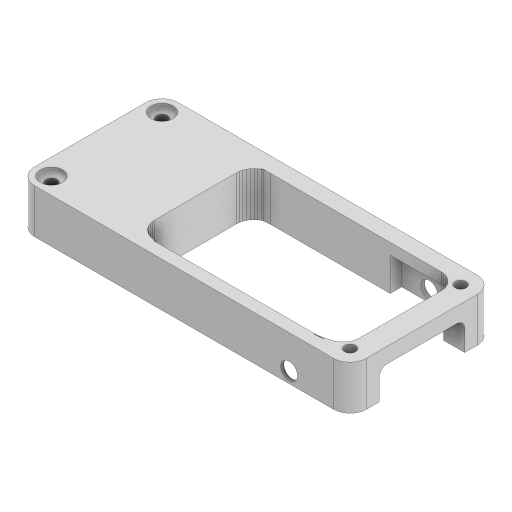
# Autodesk Inventor part: atas
Saved by Autodesk Inventor 2023 (Build 270158000, 158)
## iProperties
Created: 2025-11-27
Part Number: atas
Material: Generic
Document SubType Name: Modeling
Designer: dinoo
Density: 1 g/cm^3
Appearance: Default
Author: dinoo
Autodesk Inventor part; units mm, degrees
ref_plane "YZ Plane" through (0, 0, 0) normal (1, 0, 0) x (0, 1, 0)
ref_plane "XZ Plane" through (0, 0, 0) normal (0, 1, 0) x (-1, 0, 0)
ref_plane "XY Plane" through (0, 0, 0) normal (0, 0, 1) x (1, 0, 0)
sketch "Sketch1" plane through (0, 0, 0) normal (0, 1, 0) x (-1, 0, 0)
  circle A0 centre (50.1877, 0.0488) radius 1
  circle A1 centre (-3.8123, 20.0488) radius 1
  circle A2 centre (50.1877, 20.0488) radius 1
  circle A3 centre (-3.8123, 0.0488) radius 1
  arc A4 (53.1877, 20.0488) -> (50.1877, 23.0488) centre (50.1877, 20.0488) ccw
  line L0 (50.1877, 23.0488) -> (-3.8123, 23.0488)
  arc A5 (-3.8123, 23.0488) -> (-6.8123, 20.0488) centre (-3.8123, 20.0488) ccw
  line L1 (-6.8123, 20.0488) -> (-6.8123, 0.0488)
  arc A6 (-6.8123, 0.0488) -> (-3.8123, -2.9512) centre (-3.8123, 0.0488) ccw
  line L2 (-3.8123, -2.9512) -> (50.1877, -2.9512)
  arc A7 (50.1877, -2.9512) -> (53.1877, 0.0488) centre (50.1877, 0.0488) ccw
  line L3 (53.1877, 0.0488) -> (53.1877, 20.0488)
  line L4 (-2.6184, 2.7963) -> (-2.5855, 2.3799)
  line L5 (-2.5855, 2.3799) -> (-2.4895, 1.9806)
  line L6 (-2.4895, 1.9806) -> (-2.3323, 1.6012)
  line L7 (-2.3323, 1.6012) -> (-2.1176, 1.2511)
  line L8 (-2.1176, 1.2511) -> (-1.8508, 0.9389)
  line L9 (-1.8508, 0.9389) -> (-1.5385, 0.6723)
  line L10 (-1.5385, 0.6723) -> (-1.1883, 0.4578)
  line L11 (-1.1883, 0.4578) -> (-0.8088, 0.3008)
  line L12 (-0.8088, 0.3008) -> (-0.4112, 0.2055)
  line L13 (-0.4112, 0.2055) -> (0.0053, 0.181)
  line L14 (0.0053, 0.181) -> (30.79, 0.181)
  line L15 (30.79, 0.181) -> (32.3493, 0.3042)
  line L16 (32.3493, 0.3042) -> (31.6548, 0.1372)
  line L17 (31.6548, 0.1372) -> (32.0605, 0.3054)
  line L18 (32.0605, 0.3054) -> (32.4348, 0.535)
  line L19 (32.4348, 0.535) -> (32.7687, 0.8203)
  line L20 (32.7687, 0.8203) -> (33.0538, 1.1543)
  line L21 (33.0538, 1.1543) -> (33.2832, 1.5288)
  line L22 (33.2832, 1.5288) -> (33.4511, 1.9345)
  line L23 (33.4511, 1.9345) -> (33.5535, 2.3616)
  line L24 (33.5535, 2.3616) -> (33.5792, 2.7994)
  line L25 (33.5792, 2.7994) -> (33.5837, 17.5394)
  line L26 (33.5837, 17.5394) -> (33.5491, 17.9772)
  line L27 (33.5491, 17.9772) -> (33.4465, 18.4042)
  line L28 (33.4465, 18.4042) -> (33.2783, 18.8099)
  line L29 (33.2783, 18.8099) -> (33.0488, 19.1843)
  line L30 (33.0488, 19.1843) -> (32.7635, 19.5181)
  line L31 (32.7635, 19.5181) -> (32.4294, 19.8032)
  line L32 (32.4294, 19.8032) -> (32.0549, 20.0326)
  line L33 (32.0549, 20.0326) -> (31.6492, 20.2005)
  line L34 (31.6492, 20.2005) -> (30.2225, 20.5426)
  line L35 (30.2225, 20.5426) -> (30.7843, 20.5096)
  line L36 (30.7843, 20.5096) -> (0.0014, 20.5096)
  line L37 (0.0014, 20.5096) -> (1.8279, 20.6539)
  line L38 (1.8279, 20.6539) -> (-0.8143, 20.0188)
  line L39 (-0.8143, 20.0188) -> (-1.1937, 19.8615)
  line L40 (-1.1937, 19.8615) -> (-1.5438, 19.6468)
  line L41 (-1.5438, 19.6468) -> (-1.856, 19.38)
  line L42 (-1.856, 19.38) -> (-2.1226, 19.0677)
  line L43 (-2.1226, 19.0677) -> (-2.3371, 18.7175)
  line L44 (-2.3371, 18.7175) -> (-2.4941, 18.338)
  line L45 (-2.4941, 18.338) -> (-2.5895, 17.9404)
  line L46 (-2.5895, 17.9404) -> (-2.6139, 17.5239)
  line L47 (-2.6139, 17.5239) -> (-2.6184, 2.7963)
  circle A8 centre (-0.3906, 1.9999) radius 1.125
  circle A9 centre (3.3955, 0.901) radius 0.35
  line L48 (-1.826, 5.5906) -> (-1.026, 5.5908)
  arc A10 (-1.8262, 6.0906) -> (-1.826, 5.5906) centre (-1.8261, 5.8406) ccw
  line L49 (-1.0262, 6.0908) -> (-1.8262, 6.0906)
  arc A11 (-1.026, 5.5908) -> (-1.0262, 6.0908) centre (-1.0261, 5.8408) ccw
  line L50 (2.154, 5.5917) -> (3.3539, 5.592)
  arc A12 (2.1538, 6.0917) -> (2.154, 5.5917) centre (2.1539, 5.8417) ccw
  line L51 (3.3538, 6.092) -> (2.1538, 6.0917)
  arc A13 (3.3539, 5.592) -> (3.3538, 6.092) centre (3.3539, 5.842) ccw
  circle A14 centre (5.0955, 0.9015) radius 0.35
  circle A15 centre (8.525, 1.2724) radius 0.5
  line L52 (10.5172, 4.4875) -> (10.0672, 4.4874)
  arc A16 (10.5174, 3.9375) -> (10.5172, 4.4875) centre (10.5173, 4.2125) ccw
  line L53 (10.0674, 3.9374) -> (10.5174, 3.9375)
  arc A17 (10.0672, 4.4874) -> (10.0674, 3.9374) centre (10.0673, 4.2124) ccw
  circle A18 centre (11.065, 1.2731) radius 0.5
  circle A19 centre (2.2518, 13.0567) radius 0.381
  circle A20 centre (2.2535, 7.2768) radius 0.381
  line L54 (-1.8284, 14.2406) -> (-1.0285, 14.2408)
  arc A21 (-1.8286, 14.7406) -> (-1.8284, 14.2406) centre (-1.8285, 14.4906) ccw
  line L55 (-1.0286, 14.7408) -> (-1.8286, 14.7406)
  arc A22 (-1.0285, 14.2408) -> (-1.0286, 14.7408) centre (-1.0285, 14.4908) ccw
  circle A23 centre (-0.3951, 18.3199) radius 1.125
  line L56 (2.1515, 14.2417) -> (3.3515, 14.242)
  arc A24 (2.1514, 14.7417) -> (2.1515, 14.2417) centre (2.1515, 14.4917) ccw
  line L57 (3.3514, 14.742) -> (2.1514, 14.7417)
  arc A25 (3.3515, 14.242) -> (3.3514, 14.742) centre (3.3515, 14.492) ccw
  line L58 (10.5139, 16.3375) -> (10.0639, 16.3374)
  arc A26 (10.5141, 15.7875) -> (10.5139, 16.3375) centre (10.514, 16.0625) ccw
  line L59 (10.0641, 15.7874) -> (10.5141, 15.7875)
  arc A27 (10.0639, 16.3374) -> (10.0641, 15.7874) centre (10.064, 16.0624) ccw
  circle A28 centre (3.3904, 19.4208) radius 0.35
  circle A29 centre (8.52, 19.0524) radius 0.5
  circle A30 centre (5.0904, 19.4213) radius 0.35
  circle A31 centre (18.685, 1.2752) radius 0.5
  circle A32 centre (21.225, 1.2759) radius 0.5
  circle A33 centre (13.605, 1.2738) radius 0.5
  circle A34 centre (16.145, 1.2745) radius 0.5
  circle A35 centre (23.765, 1.2767) radius 0.5
  circle A36 centre (26.305, 1.2774) radius 0.5
  circle A37 centre (28.845, 1.2781) radius 0.5
  circle A38 centre (31.609, 3.5289) radius 1.125
  circle A39 centre (16.14, 19.0545) radius 0.5
  circle A40 centre (18.68, 19.0552) radius 0.5
  circle A41 centre (11.06, 19.0531) radius 0.5
  circle A42 centre (13.6, 19.0538) radius 0.5
  circle A43 centre (28.84, 19.0581) radius 0.5
  circle A44 centre (31.6053, 16.8088) radius 1.125
  circle A45 centre (21.22, 19.0559) radius 0.5
  circle A46 centre (26.3, 19.0574) radius 0.5
  circle A47 centre (23.76, 19.0567) radius 0.5
  line L60 (33.9837, 17.5551) -> (33.9792, 2.7876)
  line L61 (33.9792, 2.7876) -> (33.9507, 2.3028)
  line L62 (33.9507, 2.3028) -> (33.8327, 1.8107)
  line L63 (33.8327, 1.8107) -> (33.6407, 1.3467)
  line L64 (33.6407, 1.3467) -> (33.3785, 0.9185)
  line L65 (33.3785, 0.9185) -> (33.0525, 0.5366)
  line L66 (33.0525, 0.5366) -> (32.6708, 0.2104)
  line L67 (32.6708, 0.2104) -> (32.2427, -0.0521)
  line L68 (32.2427, -0.0521) -> (31.7789, -0.2443)
  line L69 (31.7789, -0.2443) -> (32.4121, -0.0921)
  line L70 (32.4121, -0.0921) -> (30.8058, -0.219)
  line L71 (30.8058, -0.219) -> (-0.0064, -0.219)
  line L72 (-0.0064, -0.219) -> (-0.47, -0.1918)
  line L73 (-0.47, -0.1918) -> (-0.9327, -0.0808)
  line L74 (-0.9327, -0.0808) -> (-1.3703, 0.1003)
  line L75 (-1.3703, 0.1003) -> (-1.7742, 0.3476)
  line L76 (-1.7742, 0.3476) -> (-2.1344, 0.6551)
  line L77 (-2.1344, 0.6551) -> (-2.4421, 1.0152)
  line L78 (-2.4421, 1.0152) -> (-2.6897, 1.419)
  line L79 (-2.6897, 1.419) -> (-2.8711, 1.8565)
  line L80 (-2.8711, 1.8565) -> (-2.9818, 2.317)
  line L81 (-2.9818, 2.317) -> (-3.0184, 2.7806)
  line L82 (-3.0184, 2.7806) -> (-3.0139, 17.5357)
  line L83 (-3.0139, 17.5357) -> (-2.9867, 17.9992)
  line L84 (-2.9867, 17.9992) -> (-2.8758, 18.4619)
  line L85 (-2.8758, 18.4619) -> (-2.6946, 18.8995)
  line L86 (-2.6946, 18.8995) -> (-2.4473, 19.3034)
  line L87 (-2.4473, 19.3034) -> (-2.1398, 19.6637)
  line L88 (-2.1398, 19.6637) -> (-1.7797, 19.9714)
  line L89 (-1.7797, 19.9714) -> (-1.3759, 20.2189)
  line L90 (-1.3759, 20.2189) -> (-0.9384, 20.4003)
  line L91 (-0.9384, 20.4003) -> (1.765, 21.0502)
  line L92 (1.765, 21.0502) -> (-0.0143, 20.9096)
  line L93 (-0.0143, 20.9096) -> (30.796, 20.9096)
  line L94 (30.796, 20.9096) -> (30.2813, 20.9398)
  line L95 (30.2813, 20.9398) -> (31.773, 20.5822)
  line L96 (31.773, 20.5822) -> (32.237, 20.3901)
  line L97 (32.237, 20.3901) -> (32.6652, 20.1279)
  line L98 (32.6652, 20.1279) -> (33.0471, 19.8019)
  line L99 (33.0471, 19.8019) -> (33.3733, 19.4202)
  line L100 (33.3733, 19.4202) -> (33.6358, 18.9921)
  line L101 (33.6358, 18.9921) -> (33.8281, 18.5283)
  line L102 (33.8281, 18.5283) -> (33.9454, 18.0401)
  line L103 (33.9454, 18.0401) -> (33.9837, 17.5551)
  point P0 (0, 0)
  point P1 (-6.8123, -2.9512)
  point P2 (-2.79, -0.0008)
  point P3 (31.9888, 0.2757)
  point P4 (1.2278, 20.5096)
  point P5 (30.3601, 20.5096)
  point P6 (32.0835, -0.1181)
  point P7 (1.1804, 20.9096)
  point P8 (30.4074, 20.9096)
  dimension "d0" = 20.3286
  dimension "d1" = 0.017
  dimension "d4" = 0.4
  constraints: 208 end point, 48 centre point, 32 point on circle, 43 other
  measures "d0" distance between parallel lines of L14 L36
  measures "d1" angle of L47 L1
  measures "d4" distance between parallel lines of L25 L60
extrude "Extrusion1" add sketch "Sketch1" along normal blind 8 contours L3 A7 L2 A6 L1 A5 L0 A4
sketch "Sketch2" plane through (6.8123, 0, 20.0488) normal (1, 0, 0) x (0, 0, -1)
  line L0 (0, 0) -> (20, 0) projected
  line L1 (20, 0) -> (20, 8) projected
  line L2 (0, 8) -> (20, 8) projected
  line L3 (0, 0) -> (0, 8) projected
  line L4 (14, -1.8137) -> (6, -1.8137)
  line L5 (6, -1.8137) -> (6, 3)
  line L6 (6, 3) -> (14, 3)
  line L7 (14, 3) -> (14, -1.8137)
  line L8 (14, -1.8137) -> (6, 3) construction
  line L9 (6, -1.8137) -> (14, 3) construction
  line L10 (15, 4) -> (5, 4)
  line L11 (5, 4) -> (5, -2.8137)
  line L12 (5, -2.8137) -> (15, -2.8137)
  line L13 (15, -2.8137) -> (15, 4)
  line L14 (14.6, 3.6) -> (5.4, 3.6)
  line L15 (5.4, 3.6) -> (5.4, -2.4137)
  line L16 (5.4, -2.4137) -> (14.6, -2.4137)
  line L17 (14.6, -2.4137) -> (14.6, 3.6)
  line L18 (4.5096, -3.3041) -> (4.5096, 4.4904)
  line L19 (4.5096, 4.4904) -> (15.4904, 4.4904)
  line L20 (15.4904, 4.4904) -> (15.4904, -3.3041)
  line L21 (15.4904, -3.3041) -> (4.5096, -3.3041)
  line L22 (17.7531, -4.072) -> (2.2469, -4.072)
  line L23 (2.2469, -4.072) -> (2.2469, 5.2583)
  line L24 (2.2469, 5.2583) -> (17.7531, 5.2583)
  line L25 (17.7531, 5.2583) -> (17.7531, -4.072)
  line L26 (17.7531, -4.072) -> (2.2469, 5.2583) construction
  line L27 (2.2469, -4.072) -> (17.7531, 5.2583) construction
  point P0 (20.0488, 0)
  point P1 (10, 0.5932)
  point P2 (6, 0)
  point P3 (14, 0)
  point P4 (14.6, 0)
  point P5 (5.4, 0)
  point P6 (15, 0)
  point P7 (15.4904, 0)
  point P8 (4.5096, 0)
  point P9 (5, 0)
  point P10 (17.7531, 0)
  point P11 (2.2469, 0)
  dimension "d7" = 1
  dimension "d8" = 0.6
  constraints: 48 end point, 10 parallel, 5 perpendicular, 4 midpoint, 2 horizontal, 9 other
  measures "d7" distance between parallel lines of L6 L10
  measures "d8" distance between parallel lines of L6 L14
extrude "Extrusion2" cut sketch "Sketch2" against normal blind 13.75 contours L23 L24 L25 L0 L20 L19 L18 | L18 L19 L20 L0 L13 L10 L11 | L11 L10 L13 L0 L17 L14 L15 | L0 L15 L16 L17 L13 L12 L11 | L15 L14 L17 L0 L7 L6 L5 | L0 L5 L4 L7 L17 L16 L15 | L5 L6 L7 L0 | L0 L7 L4 L5
fillet "Fillet1" radius 1.5 2 edges at (4.9053, 5.2583, 17.8019) (4.8945, 5.2583, 2.2957)
fillet "Fillet2" radius 1 2 edges at (-49.1877, 8, 20.0488) (-49.1877, 8, 0.0488) inverted yes
sketch "Sketch3" plane through (3.8123, 0, -2.9512) normal (0, 0, -1) x (-1, 0, 0)
  circle A0 centre (8, 2) radius 1.5
  point P0 (3.8123, 0)
  dimension "d11" = 3
  constraints: 1 centre point
  measures "d11" diameter of A0
extrude "Extrusion3" cut sketch "Sketch3" against normal blind 31.25
sketch "Sketch4" plane through (-1.1804, 8, 20.9096) normal (0, 0, -1) x (-1, 0, 0)
  line L0 (7.1098, -2.8918) -> (-1.0952, -2.8918)
  line L1 (-1.0952, -2.8918) -> (-1.0952, -9.1082)
  line L2 (-1.0952, -9.1082) -> (7.1098, -9.1082)
  line L3 (7.1098, -9.1082) -> (7.1098, -2.8918)
  circle A0 centre (3.0073, -6) radius 1.5 projected
  line L4 (7.1098, -2.8918) -> (-1.0952, -9.1082) construction
  line L5 (-1.0952, -2.8918) -> (7.1098, -9.1082) construction
  line L6 (8, -2.0016) -> (-1.9854, -2.0016)
  line L7 (-1.9854, -2.0016) -> (-1.9854, -9.9984)
  line L8 (-1.9854, -9.9984) -> (8, -9.9984)
  line L9 (8, -9.9984) -> (8, -2.0016)
  point P0 (-1.1804, -8)
  point P1 (3.0073, -8)
  constraints: 20 end point, 4 parallel, 2 midpoint, 2 perpendicular, 1 horizontal, 1 vertical alignment, 3 other
extrude "Extrusion4" cut sketch "Sketch4" along normal blind 23.2 and the other way blind 1.6 contours L3 L2 L1 L0 | A0 | L9 L8 L7 L6
body "Solid1"
